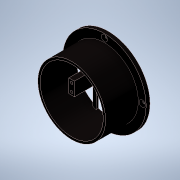
# Autodesk Inventor part: Podstawa1
Saved by Autodesk Inventor 2022 (Build 260153000, 153)
## iProperties
Created: 2023-11-10
Part Number: Podstawa1
Material: Ogólny
Document SubType Name: Modeling
Designer: nosal
Density: 1 g/cm^3
Appearance: Domyślna
Author: nosal
Autodesk Inventor part; units mm, degrees
ref_plane "YZ Plane" through (0, 0, 0) normal (1, 0, 0) x (0, 1, 0)
ref_plane "XZ Plane" through (0, 0, 0) normal (0, 1, 0) x (-1, 0, 0)
ref_plane "XY Plane" through (0, 0, 0) normal (0, 0, 1) x (1, 0, 0)
sketch "Szkic1" plane through (0, 0, 0) normal (0, 0, 1) x (1, 0, 0)
  circle A0 centre (0, 0) radius 40
  circle A1 centre (0, 0) radius 53
  dimension "d0" = 80
  dimension "d1" = 13
  constraints: 2 centre point, 1 coincident
  measures "d0" diameter of A0
  measures "d1" radial gap between concentric circles of A0 A1
extrude "Wyciągnięcie proste1" add sketch "Szkic1" along normal blind 5
sketch "Szkic2" plane through (0, 0, 5) normal (0, 0, 1) x (1, 0, 0)
  circle A0 centre (0, 0) radius 40 projected
  circle A1 centre (0, 0) radius 43
  dimension "d4" = 3
  constraints: 1 centre point
  measures "d4" radial gap between concentric circles of A0 A1
extrude "Wyciągnięcie proste2" add sketch "Szkic2" along normal blind 41.5
sketch "Szkic3" plane through (0, 0, 5) normal (0, 0, 1) x (1, 0, 0)
  circle A0 centre (0, 0) radius 43 projected
  line L0 (0, 43) -> (0, 53)
  circle A1 centre (0, 0) radius 53 projected
  line L1 (43, 0) -> (53, 0)
  line L2 (0, -43) -> (0, -53)
  line L3 (-43, 0) -> (-53, 0)
  point P0 (0, 48)
  point P1 (-48, 0)
  point P2 (0, -48)
  point P3 (48, 0)
  constraints: 8 end point, 8 point on circle, 4 midpoint, 1 horizontal, 1 perpendicular, 1 point on line, 1 vertical
hole "Otwór1" at (0, 48, 5) at (-48, 0, 5) at (0, -48, 5) at (48, 0, 5) direction (0, 0, -1) diameter 3.242 end through all countersink diameter 8 countersink angle 90 thread size "M4x0.7" designation "M4" class "6H" standard "GB Metric profile"
sketch "Szkic8" plane through (0, 0, 0) normal (0, 0, -1) x (-1, 0, 0)
  circle A0 centre (0, 0) radius 10.75
  line L0 (0, 0) -> (17, 0)
  line L1 (17, 0) -> (14.59, 0)
  line L2 (14.59, 0) -> (14.59, 5)
  line L3 (14.59, 0) -> (14.59, -5)
  circle A1 centre (14.59, 5) radius 1.621
  circle A2 centre (14.59, -5) radius 1.621
  line L4 (14.59, 5) -> (-35.19, 5)
  line L5 (14.59, -5) -> (-35.19, -5)
  circle A3 centre (-35.19, 5) radius 1.621
  circle A4 centre (-35.19, -5) radius 1.621
  line L6 (-33.569, -5) -> (-31.569, -5)
  line L7 (-31.569, -5) -> (-31.569, 5)
  line L8 (-35.19, 6.621) -> (-35.19, 8.621)
  line L9 (-35.19, 8.621) -> (-31.569, 8.621)
  line L10 (-31.569, 8.621) -> (-31.569, 5)
  line L11 (-36.811, 5) -> (-38.811, 5)
  line L12 (-35.19, -6.621) -> (-35.19, -8.621)
  line L13 (-35.19, -8.621) -> (-31.569, -8.621)
  line L14 (-31.569, -8.621) -> (-31.569, -5)
  line L15 (-35.19, -8.621) -> (-38.811, -8.621)
  line L16 (-38.811, 5) -> (-38.811, 8.621)
  line L17 (-38.811, 8.621) -> (-35.19, 8.621)
  line L18 (12.969, -5) -> (10.969, -5)
  line L19 (14.59, -6.621) -> (14.59, -8.621)
  line L20 (10.969, -5) -> (10.969, -8.621)
  line L21 (10.969, -8.621) -> (14.59, -8.621)
  line L22 (14.59, 6.621) -> (14.59, 8.621)
  line L23 (14.59, 8.621) -> (10.969, 8.621)
  line L24 (10.969, 8.621) -> (10.969, -5)
  line L25 (16.211, -5) -> (18.211, -5)
  line L26 (14.59, -8.621) -> (18.211, -8.621)
  line L27 (18.211, -8.621) -> (18.211, 8.621)
  line L28 (18.211, 8.621) -> (14.59, 8.621)
  circle A5 centre (0, 0) radius 40 projected
  line L29 (-38.811, -8.621) -> (-39.0599, -8.621)
  line L30 (-38.811, 8.621) -> (-39.0599, 8.621)
  line L31 (-31.569, 8.621) -> (-30.569, 8.621)
  line L32 (-30.569, 8.621) -> (-30.569, -8.621)
  line L33 (-30.569, -8.621) -> (-31.569, -8.621)
  dimension "d59" = 3.242
  dimension "d54" = 21.5
  dimension "d55" = 17
  dimension "d56" = 2.41
  dimension "d57" = 5
  dimension "d58" = 5
  dimension "d60" = 3.242
  dimension "d61" = 49.78
  dimension "d62" = 3.242
  dimension "d63" = 3.242
  dimension "d64" = 2
  dimension "d66" = 2
  dimension "d67" = 2
  dimension "d68" = 2
  dimension "d69" = 2
  dimension "d70" = 2
  dimension "d71" = 2
  dimension "d74" = 49.78
  dimension "d87" = 1
  constraints: 68 end point, 13 perpendicular, 9 point on circle, 8 horizontal, 6 point on line, 6 vertical, 5 coincident, 4 centre point, 2 collinear, 2 parallel, 1 vertical alignment, 2 other
  measures "d54" diameter of A0
  measures "d55" distance of L0.start L0.end
  measures "d56" distance of L0.end L1.end
  measures "d57" distance of L1.end L2.end
  measures "d58" distance of L1.end L3.end
  measures "d60" diameter of A2
  measures "d61" distance of L4.start L4.end
  measures "d62" diameter of A3
  measures "d63" diameter of A4
  measures "d64" distance of L6.start L6.end
  measures "d66" distance of L8.start L8.end
  measures "d67" distance of L11.end L11.start
  measures "d68" distance of L12.start L12.end
  measures "d69" distance of L18.start L18.end
  measures "d70" distance of L19.start L19.end
  measures "d71" distance of L25.start L25.end
  measures "d74" distance of L5.end L3.end
  measures "d87" distance of L9.end L31.end
extrude "Wyciągnięcie proste6" add sketch "Szkic8" against normal blind 32 contours L24 L4 A1 L2 L0 | L0 L3 A2 L5 L24 | L24 L23 L22 A1 L4 | L5 A2 L19 L21 L20 | L2 A1 L22 L28 L27 L25 A2 L3 | L7 L5 A4 L12 L15 L29 A5 L30 L16 L11 A3 L4 | L4 A3 L8 L9 L10 | L14 L13 L12 A4 L5 | A2 L25 L27 L26 L19 | A3 L11 L16 L17 L8
sketch "Szkic9" plane through (0, 0, 0) normal (0, 0, -1) x (-1, 0, 0)
  line L0 (11.0032, 0) -> (10.969, -1.9997)
  line L1 (10.969, -8.621) -> (10.969, 8.621) projected
  line L2 (10.969, -1.9997) -> (10.969, 2.0003)
  line L3 (10.969, 2.0003) -> (-31.569, 2.0003)
  line L4 (-31.569, -8.621) -> (-31.569, 8.621) projected
  line L5 (10.969, -1.9997) -> (-31.569, -1.9997)
  circle A0 centre (14.59, -5) radius 1.621 projected
  line L6 (14.59, -5) -> (14.59, -8.621)
  line L7 (18.211, -8.621) -> (10.969, -8.621) projected
  line L8 (14.59, -8.621) -> (12.59, -8.621)
  line L9 (12.59, -8.621) -> (16.59, -8.621)
  line L10 (16.59, -8.621) -> (16.59, -36.3974)
  arc A1 (-39.0599, -8.621) -> (-39.0599, 8.621) centre (0, 0) ccw projected
  line L11 (12.59, -8.621) -> (12.59, -37.967)
  line L12 (10.969, 8.621) -> (18.211, 8.621) projected
  line L13 (12.59, 8.621) -> (12.59, 45.8086)
  line L14 (12.59, 8.621) -> (49.7776, 8.621) construction
  line L15 (16.59, 8.621) -> (16.59, 43)
  point P0 (16.59, 36.3974)
  point P1 (12.59, 37.967)
  dimension "d75" = 2
  dimension "d76" = 4
  dimension "d77" = 2
  dimension "d78" = 4
  dimension "d79" = 90
  constraints: 24 end point, 6 point on line, 4 perpendicular, 2 horizontal, 2 point on circle, 2 vertical, 1 midpoint
  measures "d75" distance of L0.start L0.end
  measures "d76" distance of L0.end L2.end
  measures "d77" distance of L6.end L8.end
  measures "d78" distance of L8.end L9.end
  measures "d79" angle of L14 L13
extrude "Wyciągnięcie proste7" add sketch "Szkic9" against normal blind 3 contours L5 L4 L3 L1 | L7 L10 A1 L11 | L13 A1 L15 L12
equation "\"d62\" = d59"
equation "\"d63\" = d60"
equation "\"d74\" = d61"
